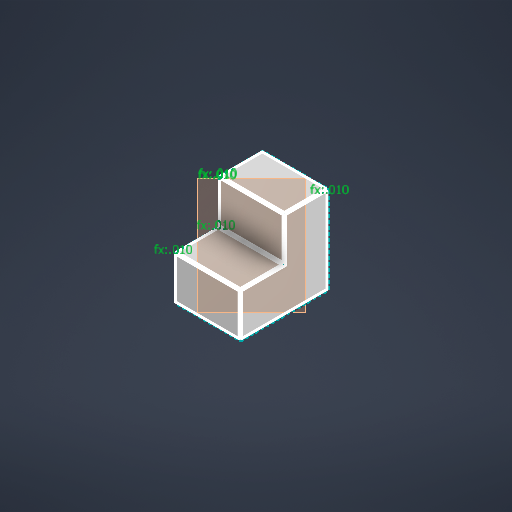
# Autodesk Inventor part: iso
Saved by Autodesk Inventor 2025.1 (Build 291241000, 241)
## iProperties
Created: 2025-06-16
Part Number: iso
Material: Generic
Document SubType Name: Modeling
Designer: riters
Density: 1 g/cm^3
Appearance: Default
Author: riters
Autodesk Inventor part; units mm, degrees
ref_plane "YZ Plane" through (0, 0, 0) normal (1, 0, 0) x (0, 1, 0)
ref_plane "XZ Plane" through (0, 0, 0) normal (0, 1, 0) x (-1, 0, 0)
ref_plane "XY Plane" through (0, 0, 0) normal (0, 0, 1) x (1, 0, 0)
sketch "Sketch1" plane through (0, 0, 0) normal (1, 0, 0) x (0, 1, 0)
  line L0 (-12.7, 12.7) -> (0, 12.7)
  line L1 (12.7, 0) -> (12.7, -12.7)
  line L2 (12.7, -12.7) -> (-12.7, -12.7)
  line L3 (-12.7, -12.7) -> (-12.7, 12.7)
  line L4 (-12.7, 12.7) -> (12.7, -12.7) construction
  line L5 (0, 0) -> (-12.7, -12.7) construction
  line L6 (0, 0) -> (12.7, 0)
  line L7 (0, 12.7) -> (0, 0)
  line L8 (12.7, 0) -> (0, 0)
  dimension "d0" = 25.4
  constraints: 18 end point, 2 horizontal, 2 midpoint, 2 parallel, 2 perpendicular, 1 collinear, 1 point on line, 1 vertical
  measures "d0" distance of L1.end L2.end
extrude "Extrusion1" add sketch "Sketch1" along normal mid plane 19.05
ref_plane "Work Plane2" through (29.3294, 29.3294, 29.3294) normal (0.5774, 0.5774, 0.5774) x (0.7071, 0, -0.7071)
ref_plane "Work Plane1" through (0, 0, 0) normal (0.5774, 0.5774, 0.5774) x (0.7071, 0, -0.7071)
sketch "Sketch2" plane through (29.3294, 29.3294, 29.3294) normal (0.5774, 0.5774, 0.5774) x (0.7071, 0, -0.7071)
  line L0 (-6.7352, 14.2581) -> (6.7352, 6.4809) construction
  line L1 (15.7154, 11.6657) -> (6.7352, 6.4809) construction
  line L2 (2.2451, 19.4428) -> (15.7154, 11.6657) construction
  line L3 (-6.7352, 14.2581) -> (2.2451, 19.4428) construction
  line L4 (-6.7352, 3.8886) -> (6.7352, -3.8886) construction
  line L5 (6.7352, 6.4809) -> (6.7352, -3.8886) construction
  line L6 (-6.7352, 14.2581) -> (6.7352, 6.4809) construction
  line L7 (-6.7352, 3.8886) -> (-6.7352, 14.2581) construction
  line L8 (-2.2451, -9.0733) -> (-15.7154, -1.2962) construction
  line L9 (6.7352, -3.8886) -> (-2.2451, -9.0733) construction
  line L10 (-6.7352, 3.8886) -> (6.7352, -3.8886) construction
  line L11 (-15.7154, -1.2962) -> (-6.7352, 3.8886) construction
  line L12 (-15.7154, -11.6657) -> (-2.2451, -19.4428) construction
  line L13 (-2.2451, -9.0733) -> (-2.2451, -19.4428) construction
  line L14 (-2.2451, -9.0733) -> (-15.7154, -1.2962) construction
  line L15 (-15.7154, -11.6657) -> (-15.7154, -1.2962) construction
  line L16 (-2.2451, -9.0733) -> (-2.2451, -19.4428) construction
  line L17 (-2.2451, -19.4428) -> (15.7154, -9.0733) construction
  line L18 (15.7154, -9.0733) -> (15.7154, 11.6657) construction
  line L19 (15.7154, 11.6657) -> (6.7352, 6.4809) construction
  line L20 (6.7352, 6.4809) -> (6.7352, -3.8886) construction
  line L21 (6.7352, -3.8886) -> (-2.2451, -9.0733) construction
  line L22 (6.7352, 6.7742) -> (-6.2272, 14.2581)
  line L23 (-6.2272, 14.2581) -> (2.2451, 19.1495)
  line L24 (2.2451, 19.1495) -> (15.2074, 11.6657)
  line L25 (15.2074, 11.6657) -> (6.7352, 6.7742)
  line L26 (-6.4812, 13.8181) -> (6.4812, 6.3343)
  line L27 (6.4812, 6.3343) -> (6.4812, -3.4486)
  line L28 (6.4812, -3.4486) -> (-6.4812, 4.0352)
  line L29 (-6.4812, 4.0352) -> (-6.4812, 13.8181)
  line L30 (-6.7352, 3.5953) -> (6.2272, -3.8886)
  line L31 (6.2272, -3.8886) -> (-2.2451, -8.78)
  line L32 (-2.2451, -8.78) -> (-15.2074, -1.2962)
  line L33 (-15.2074, -1.2962) -> (-6.7352, 3.5953)
  line L34 (-15.4614, -1.7361) -> (-2.4991, -9.22)
  line L35 (-2.4991, -9.22) -> (-2.4991, -19.0029)
  line L36 (-2.4991, -19.0029) -> (-15.4614, -11.519)
  line L37 (-15.4614, -11.519) -> (-15.4614, -1.7361)
  line L38 (15.4614, 11.2258) -> (15.4614, -8.9267)
  line L39 (15.4614, -8.9267) -> (-1.9911, -19.0029)
  line L40 (-1.9911, -19.0029) -> (-1.9911, -9.22)
  line L41 (-1.9911, -9.22) -> (6.9892, -4.0352)
  line L42 (6.9892, -4.0352) -> (6.9892, 6.3343)
  line L43 (6.9892, 6.3343) -> (15.4614, 11.2258)
  point P0 (0, 0)
  dimension "d5" = 0.254
  dimension "d6" = 0.254
  dimension "d7" = 0.254
  dimension "d8" = 0.254
  dimension "d9" = 0.254
  constraints: 44 end point, 17 other
  measures "d5" distance between parallel lines of L22 L0
  measures "d6" distance between parallel lines of L0 L26
  measures "d7" distance between parallel lines of L43 L1
  measures "d8" distance between parallel lines of L4 L30
  measures "d9" distance between parallel lines of L8 L34
equation "\"d5\" = 0.5 * spacing"
equation "\"d6\" = 0.5 * spacing"
equation "\"d7\" = 0.5 * spacing"
equation "\"d8\" = 0.5 * spacing"
equation "\"d9\" = 0.5 * spacing"
equation "\"spacing\" = 0.508"
body "Solid1"
